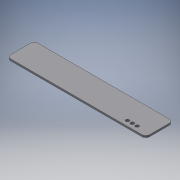
# Autodesk Inventor part: case-front
Saved by Autodesk Inventor 2017 (Build 210142000, 142)
## iProperties
Created: 2020-10-01
Part Number: case-front
Material: Generic
Document SubType Name: Modeling
Designer: jferner
Density: 1 g/cm^3
Appearance: Default
Author: jferner
Autodesk Inventor part; units mm, degrees
ref_plane "YZ Plane" through (0, 0, 0) normal (1, 0, 0) x (0, 1, 0)
ref_plane "XZ Plane" through (0, 0, 0) normal (0, 1, 0) x (-1, 0, 0)
ref_plane "XY Plane" through (0, 0, 0) normal (0, 0, 1) x (1, 0, 0)
sketch "Sketch1" plane through (0, 0, 0) normal (0, 0, 1) x (1, 0, 0)
  line L0 (4, 0) -> (144, 0)
  line L1 (148, 4) -> (148, 25)
  line L2 (144, 29) -> (4, 29)
  line L3 (0, 25) -> (0, 4)
  arc A0 (0, 4) -> (4, 0) centre (4, 4) ccw
  arc A1 (144, 0) -> (148, 4) centre (144, 4) ccw
  arc A2 (148, 25) -> (144, 29) centre (144, 25) ccw
  arc A3 (4, 29) -> (0, 25) centre (4, 25) ccw
  point P0 (0, 0)
  point P1 (148, 29)
  point P2 (148, 0)
  point P3 (0, 29)
  dimension "d2" = 4
  dimension "d3" = 148
  dimension "d4" = 29
  constraints: 8 end point, 8 point on circle, 8 point on line, 8 tangent, 4 centre point, 3 equal radius, 2 parallel, 1 horizontal, 1 perpendicular
  measures "d2" radius of A0
  measures "d3" distance between parallel lines of L1 L3
  measures "d4" distance between parallel lines of L2 L0
extrude "Extrusion1" add sketch "Sketch1" along normal blind 2
sketch "Sketch2" plane through (0, 0, 2) normal (0, 0, 1) x (1, 0, 0)
  circle A0 centre (123.3, 5.3) radius 1.897
  line L0 (3.231, -4.8492) -> (37.2409, -4.8492)
  circle A1 centre (128.4, 5.3) radius 1.897
  circle A2 centre (133.5, 5.3) radius 1.897
  line L1 (4, 0) -> (144, 0) projected
  line L2 (0, 25) -> (0, 4) projected
  line L3 (148, 4) -> (148, 25) projected
  point P0 (0, 0)
  dimension "d7" = 5.1
  dimension "distanceFromTop" = 5.3
  dimension "d14" = 3.794
  dimension "distanceFromSide" = 14.5
  constraints: 3 centre point, 2 end point, 2 horizontal, 4 other
  measures "d7" distance of A0.centre A1.centre
  measures "distanceFromTop" distance from line of L1 A0.centre
  measures "d14" diameter of A0
  measures "distanceFromSide" distance from line of L3 A2.centre
extrude "Extrusion2" cut sketch "Sketch2" against normal through all
equation "\"d2\" = filletMid"
equation "\"d3\" = caseBottomWidth - thickness"
equation "\"d4\" = -thickness + 2 * caseBottomHeight - lipHeight"
equation "\"d0\" = thickness"
equation "\"d15\" = thickness"
equation "\"filletMid\" = 4"
equation "\"caseBottomWidth\" = 150"
equation "\"thickness\" = 2"
equation "\"caseBottomHeight\" = 16"
equation "\"lipHeight\" = 1"
body "Solid1"
